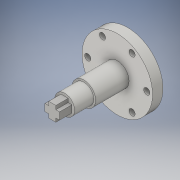
# Autodesk Inventor part: OmniWheelAxle
Saved by Autodesk Inventor 2016 (Build 200138000, 138)
## iProperties
Created: 2016-12-01
Part Number: OmniWheelAxle
Material: Generic
Document SubType Name: Modeling
Designer: Evan Phil George
Density: 1 g/cm^3
Appearance: Default
Author: Evan Phil George
Autodesk Inventor part; units mm, degrees
ref_plane "YZ Plane" through (0, 0, 0) normal (1, 0, 0) x (0, 1, 0)
ref_plane "XZ Plane" through (0, 0, 0) normal (0, 1, 0) x (-1, 0, 0)
ref_plane "XY Plane" through (0, 0, 0) normal (0, 0, 1) x (1, 0, 0)
sketch "Sketch1" plane through (0, 0, 0) normal (0, 0, 1) x (1, 0, 0)
  circle A0 centre (0, 0) radius 28.45
  dimension "d0" = 56.9
  constraints: 1 centre point, 1 coincident
  measures "d0" diameter of A0
extrude "Extrusion1" add sketch "Sketch1" along normal blind 8.4
sketch "Sketch2" plane through (0, 0, 8.4) normal (0, 0, 1) x (1, 0, 0)
  line L0 (0, 0) -> (23.85, 0)
  line L1 (0, 0) -> (11.925, 20.6547)
  line L2 (0, 0) -> (23.85, 0) construction
  line L3 (0, 0) -> (-11.925, 20.6547)
  line L4 (0, 0) -> (23.85, 0) construction
  line L5 (0, 0) -> (-23.85, 0)
  line L6 (0, 0) -> (23.85, 0) construction
  line L7 (0, 0) -> (11.925, -20.6547)
  line L8 (0, 0) -> (23.85, 0) construction
  line L9 (0, 0) -> (-11.925, -20.6547)
  line L10 (0, 0) -> (23.85, 0) construction
  circle A0 centre (23.85, 0) radius 2.5
  circle A1 centre (11.925, 20.6547) radius 2.5
  circle A2 centre (11.925, -20.6547) radius 2.5
  circle A3 centre (-11.925, -20.6547) radius 2.5
  circle A4 centre (-23.85, 0) radius 2.5
  circle A5 centre (-11.925, 20.6547) radius 2.5
  dimension "d3" = 23.85
  dimension "d4" = 23.85
  dimension "d5" = 60
  dimension "d6" = 23.85
  dimension "d7" = 120
  dimension "d8" = 23.85
  dimension "d9" = 180
  dimension "d10" = 23.85
  dimension "d11" = 60
  dimension "d12" = 23.85
  dimension "d13" = 120
  dimension "d14" = 5
  dimension "d15" = 5
  dimension "d16" = 5
  dimension "d17" = 5
  dimension "d18" = 5
  dimension "d19" = 5
  constraints: 22 end point, 7 horizontal, 6 centre point, 6 coincident, 5 equal length
  measures "d3" distance of L0.start L0.end
  measures "d4" distance of L0.start L1.end
  measures "d5" angle of L2 L1
  measures "d6" distance of L0.start L3.end
  measures "d7" angle of L4 L3
  measures "d8" distance of L0.start L5.end
  measures "d9" angle of L5 L6
  measures "d10" distance of L0.start L7.end
  measures "d11" angle of L7 L8
  measures "d12" distance of L0.start L9.end
  measures "d13" angle of L9 L10
  measures "d14" diameter of A0
  measures "d15" diameter of A1
  measures "d16" diameter of A2
  measures "d17" diameter of A3
  measures "d18" diameter of A4
  measures "d19" diameter of A5
extrude "Extrusion2" cut sketch "Sketch2" against normal blind 8.4
sketch "Sketch3" plane through (0, 0, 8.4) normal (0, 0, 1) x (1, 0, 0)
  circle A0 centre (0, 0) radius 9.5
  dimension "d22" = 19
  constraints: 1 centre point, 1 coincident
  measures "d22" diameter of A0
extrude "Extrusion3" add sketch "Sketch3" along normal blind 27
sketch "Sketch4" plane through (0, 0, 35.4) normal (0, 0, 1) x (1, 0, 0)
  circle A0 centre (0, 0) radius 8
  dimension "d25" = 16
  constraints: 1 centre point, 1 coincident
  measures "d25" diameter of A0
extrude "Extrusion4" add sketch "Sketch4" along normal blind 15.5
sketch "Sketch6" plane through (0, 0, 0) normal (0, 0, -1) x (-1, 0, 0)
  line L0 (0, 0) -> (0, 9)
  line L1 (0, 9) -> (2, 9)
  line L2 (2, 9) -> (2, 2)
  line L3 (2, 2) -> (9, 2)
  line L4 (9, 2) -> (9, -2)
  line L5 (9, -2) -> (2, -2)
  line L6 (2, -2) -> (2, -9)
  line L7 (2, -9) -> (-2, -9)
  line L8 (-2, -9) -> (-2, -2)
  line L9 (-2, -2) -> (-9, -2)
  line L10 (-9, -2) -> (-9, 2)
  line L11 (-9, 2) -> (-2, 2)
  line L12 (-2, 2) -> (-2, 9)
  line L13 (-2, 9) -> (0, 9)
  dimension "d120" = 9
  dimension "d121" = 2
  dimension "d122" = 7
  dimension "d124" = 7
  dimension "d125" = 4
  dimension "d126" = 7
  dimension "d127" = 7
  dimension "d128" = 4
  dimension "d129" = 7
  dimension "d130" = 7
  dimension "d131" = 4
  dimension "d132" = 7
  dimension "d133" = 7
  constraints: 28 end point, 7 perpendicular, 3 horizontal, 2 point on line, 1 vertical
  measures "d120" distance of L0.start L0.end
  measures "d121" distance of L0.end L1.end
  measures "d122" distance of L1.end L2.end
  measures "d124" distance of L2.end L3.end
  measures "d125" distance of L3.end L4.end
  measures "d126" distance of L4.end L5.end
  measures "d127" distance of L5.end L6.end
  measures "d128" distance of L6.end L7.end
  measures "d129" distance of L7.end L8.end
  measures "d130" distance of L8.end L9.end
  measures "d131" distance of L9.end L10.end
  measures "d132" distance of L10.end L11.end
  measures "d133" distance of L11.end L12.end
extrude "Extrusion6" cut sketch "Sketch6" against normal blind 6
sketch "Sketch7" plane through (0, 0, 6) normal (0, 0, -1) x (-1, 0, 0)
  circle A0 centre (0, 0) radius 1.5
  dimension "d91" = 3
  constraints: 1 centre point, 1 coincident
  measures "d91" diameter of A0
extrude "Extrusion7" cut sketch "Sketch7" against normal blind 5
thread "Thread3" size "M3x0.5" class "6H" standard "ANSI Metric M Profile" full length
sketch "Sketch12" plane through (0, 0, 50.9) normal (0, 0, 1) x (1, 0, 0)
  line L0 (0, 0) -> (5.9, 0)
  line L1 (5.9, 0) -> (5.9, 2.9)
  line L2 (5.9, 0) -> (5.9, -2.9)
  line L3 (5.9, 2.9) -> (2.9, 2.9)
  line L4 (2.9, 2.9) -> (2.9, 5.9)
  line L5 (5.9, -2.9) -> (2.9, -2.9)
  line L6 (2.9, -2.9) -> (2.9, -5.9)
  line L7 (2.9, -5.9) -> (-2.9, -5.9)
  line L8 (-2.9, -5.9) -> (-2.9, -2.9)
  line L9 (-2.9, -2.9) -> (-5.9, -2.9)
  line L10 (-5.9, -2.9) -> (-5.9, 2.9)
  line L11 (-5.9, 2.9) -> (-2.9, 2.9)
  line L12 (-2.9, 2.9) -> (-2.9, 5.9)
  line L13 (-2.9, 5.9) -> (2.9, 5.9)
  dimension "d221" = 5.9
  dimension "d222" = 2.9
  dimension "d223" = 2.9
  dimension "d224" = 3
  dimension "d225" = 3
  dimension "d226" = 3
  dimension "d227" = 3
  dimension "d228" = 5.8
  dimension "d229" = 3
  dimension "d230" = 3
  dimension "d231" = 5.8
  dimension "d232" = 3
  dimension "d233" = 3
  constraints: 28 end point, 5 perpendicular, 4 vertical, 2 horizontal, 2 point on line
  measures "d221" distance of L0.start L0.end
  measures "d222" distance of L0.end L1.end
  measures "d223" distance of L0.end L2.end
  measures "d224" distance of L1.end L3.end
  measures "d225" distance of L3.end L4.end
  measures "d226" distance of L2.end L5.end
  measures "d227" distance of L5.end L6.end
  measures "d228" distance of L6.end L7.end
  measures "d229" distance of L7.end L8.end
  measures "d230" distance of L8.end L9.end
  measures "d231" distance of L9.end L10.end
  measures "d232" distance of L10.end L11.end
  measures "d233" distance of L11.end L12.end
extrude "Extrusion11" add sketch "Sketch12" along normal blind 10
body "Solid1"
